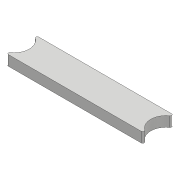
# Autodesk Inventor part: arm_0_extension_attacher
Saved by Autodesk Inventor 2018 (Build 220112000, 112)
## iProperties
Created: 2018-08-17
Part Number: arm_0_extension_attacher
Material: Generic
Document SubType Name: Modeling
Designer: Bardo91
Density: 1 g/cm^3
Appearance: Default
Author: Bardo91
Autodesk Inventor part; units mm, degrees
ref_plane "YZ Plane" through (0, 0, 0) normal (1, 0, 0) x (0, 1, 0)
ref_plane "XZ Plane" through (0, 0, 0) normal (0, 1, 0) x (-1, 0, 0)
ref_plane "XY Plane" through (0, 0, 0) normal (0, 0, 1) x (1, 0, 0)
sketch "Sketch1" plane through (0, 0, 0) normal (0, 0, 1) x (1, 0, 0)
  arc A0 (0, -30) -> (0, 30) centre (0, 0) ccw
  line L0 (0, 0) -> (300, 0)
  arc A1 (300, 30) -> (300, -30) centre (300, 0) ccw
  line L1 (300, 30) -> (0, 30)
  line L2 (300, -30) -> (0, -30)
  dimension "d6" = 60
  dimension "d7" = 300
  dimension "d8" = 60
  constraints: 6 end point, 4 point on circle, 2 centre point, 2 horizontal, 1 coincident, 1 parallel
  measures "d6" diameter of A0
  measures "d7" distance of L0.start L0.end
  measures "d8" diameter of A1
extrude "Extrusion2" add sketch "Sketch1" along normal blind 20
fillet "Fillet2" radius 3 4 edges at (300, 30, 10) (300, -30, 10) (0, -30, 10) (0, 30, 10)
body "Solid2"
